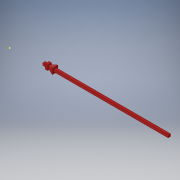
# Autodesk Inventor part: MiddleStick
Saved by Autodesk Inventor 2018.2 (Build 222227000, 227)
## iProperties
Created: 2018-04-10
Part Number: MiddleStick
Material: Generisch
Document SubType Name: Modeling
Designer: Nick Koch
Density: 1 g/cm^3
Appearance: Vorgabe
Author: Nick Koch
Autodesk Inventor part; units mm, degrees
ref_plane "YZ Plane" through (0, 0, 0) normal (1, 0, 0) x (0, 1, 0)
ref_plane "XZ Plane" through (0, 0, 0) normal (0, 1, 0) x (-1, 0, 0)
ref_plane "XY Plane" through (0, 0, 0) normal (0, 0, 1) x (1, 0, 0)
sketch "Skizze4" plane through (0, 0, 0) normal (0, 0, 1) x (1, 0, 0)
  line L0 (0, 0) -> (200, 0)
  line L1 (200, 0) -> (200, 3)
  line L2 (200, 3) -> (0, 3)
  line L3 (0, 3) -> (0, 0)
  dimension "d12" = 200
  dimension "d13" = 3
  constraints: 8 end point, 2 parallel, 1 horizontal, 1 perpendicular
  measures "d12" distance of L2.end L1.end
  measures "d13" distance of L1.end L0.end
extrude "Extrusion4" add sketch "Skizze4" along normal blind 3
sketch "Skizze5" plane through (0, 0, 3) normal (0, 0, 1) x (1, 0, 0)
  line L0 (47, 5) -> (50, 5)
  line L1 (50, 5) -> (50, -2)
  line L2 (50, -2) -> (47, -2)
  line L3 (47, -2) -> (47, 5)
  line L4 (200, 0) -> (200, 3) projected
  line L5 (0, 3) -> (0, 0) projected
  line L6 (200, 3) -> (0, 3) projected
  line L7 (0, 0) -> (200, 0) projected
  dimension "d16" = 150
  dimension "d17" = 47
  dimension "d18" = 2
  dimension "d19" = 2
  constraints: 8 end point, 2 parallel, 1 horizontal, 1 perpendicular
  measures "d16" distance between parallel lines of L4 L1
  measures "d17" distance between parallel lines of L5 L3
  measures "d18" distance between parallel lines of L0 L6
  measures "d19" distance between parallel lines of L7 L2
extrude "Extrusion5" add sketch "Skizze5" along normal blind 2 and the other way blind 5 contours L0 L1 L6 L3 | L6 L1 L7 L3 | L7 L1 L2 L3
sketch "Skizze6" plane through (0, 0, -2) normal (0, 0, -1) x (-1, 0, 0)
  point P0 (0, 0)
sketch "Skizze7" plane through (0, 0, 0) normal (0, 0, -1) x (-1, 0, 0)
  line L0 (-200, 3) -> (-50, 3) projected
  line L1 (-78, 3) -> (-50, 3)
  line L2 (-50, 3) -> (-50, 5)
  line L3 (-50, 5) -> (-78, 5)
  line L4 (-78, 5) -> (-78, 3)
  line L5 (-50, 5) -> (-48, 5)
  line L6 (-48, 5) -> (-48, 33)
  line L7 (-48, 33) -> (-50, 33)
  line L8 (-50, 33) -> (-50, 5)
  line L9 (-50, -2) -> (-50, 5) projected
  arc A0 (-50, 30) -> (-75, 5) centre (-50, 5) ccw
  arc A1 (-50, 27.2) -> (-72.2, 5) centre (-50, 5) ccw
  line L10 (-50, 5) -> (-59.1924, 14.1924)
  line L11 (-50, 5) -> (-37, 5) construction
  circle A2 centre (-59.1924, 14.1924) radius 2.5
  line L12 (-59.1924, 14.1924) -> (-50, 14.1924)
  line L13 (-59.1924, 14.1924) -> (-50, 14.1924)
  line L14 (-50, 14.1924) -> (-50, 13.3924)
  line L15 (-50, 13.3924) -> (-59.1924, 13.3924)
  line L16 (-59.1924, 13.3924) -> (-59.1924, 14.1924)
  line L17 (-50, 14.1924) -> (-59.1924, 14.1924)
  line L18 (-59.1924, 14.1924) -> (-59.1924, 14.9924)
  line L19 (-59.1924, 14.9924) -> (-50, 14.9924)
  line L20 (-50, 14.9924) -> (-50, 14.1924)
  line L21 (-50, 30) -> (-50, 27.2)
  line L22 (-75, 5) -> (-72.2, 5)
  point P0 (0, 0)
  dimension "d24" = 2
  dimension "d25" = 2
  dimension "d26" = 50
  dimension "d27" = 2.8
  dimension "d28" = 13
  dimension "d29" = 135
  dimension "d30" = 5
  dimension "d31" = 0.8
  dimension "d32" = 0.8
  dimension "d33" = 28
  dimension "d34" = 28
  constraints: 42 end point, 8 parallel, 7 perpendicular, 4 point on circle, 4 point on line, 3 centre point, 3 horizontal, 2 coincident, 1 collinear, 1 equal length, 1 vertical
  measures "d24" distance of L2.end L1.end
  measures "d25" distance of L7.end L6.end
  measures "d26" diameter of A0
  measures "d27" radial gap between concentric circles of A0 A1
  measures "d28" distance of L10.start L10.end
  measures "d29" angle of L11 L10
  measures "d30" diameter of A2
  measures "d31" distance of L12.end L14.end
  measures "d32" distance of L12.start L18.end
  measures "d33" distance of L5.end L6.end
  measures "d34" distance of L2.end L3.end
extrude "Extrusion6" add sketch "Skizze7" against normal blind 3 contours L4 L3 L2 L0 | L8 L7 L6 L5 | A0 L8 A1 L3 | L15 A2 L12 L8 | A2 L19 L18 L16 L15 L10 | L10 L15 A2 | L12 A2 L19 L8 | L15 L10 L12 A2 | L15 L16 L10 | A2 L12 L18 L19
sketch "Skizze8" plane through (0, 0, 0) normal (0, 0, -1) x (-1, 0, 0)
  arc A0 (-56.8238, 14.9924) -> (-56.8238, 13.3924) centre (-59.1924, 14.1924) ccw projected
  circle A1 centre (-59.1924, 14.1924) radius 2.5
  line L0 (-56.8238, 13.3924) -> (-50, 13.3924) projected
  line L1 (-56.8238, 13.3924) -> (-50, 13.3924)
  line L2 (-50, 13.3924) -> (-50, 14.9924)
  line L3 (-56.8238, 14.9924) -> (-50, 14.9924) projected
  line L4 (-50, 14.9924) -> (-56.8238, 14.9924)
  point P0 (0, 0)
  constraints: 6 end point, 2 perpendicular, 1 centre point, 1 coincident, 1 collinear
extrude "Extrusion7" cut sketch "Skizze8" against normal blind 0.75 contours L3 L2 L0 A1
sketch "Skizze9" plane through (0, 0, 3) normal (0, 0, 1) x (1, 0, 0)
  arc A0 (56.8238, 13.3924) -> (56.8238, 14.9924) centre (59.1924, 14.1924) ccw projected
  circle A1 centre (59.1924, 14.1924) radius 2.5
  line L0 (50, 14.9924) -> (50, 27.2) projected
  line L1 (56.8238, 14.9924) -> (50, 14.9924)
  line L2 (50, 14.9924) -> (50, 13.3924) projected
  line L3 (50, 14.9924) -> (50, 13.3924)
  line L4 (50, 13.3924) -> (56.8238, 13.3924)
  point P0 (0, 0)
  constraints: 6 end point, 2 perpendicular, 1 coincident, 1 horizontal, 3 other
extrude "Extrusion8" cut sketch "Skizze9" against normal blind 0.75 contours L4 L2 L1 A1
sketch "Skizze10" plane through (0, 0, 0) normal (0, 0, -1) x (-1, 0, 0)
  line L0 (-47, 3) -> (-42, 3)
  line L1 (-47, 3) -> (0, 3) projected
  line L2 (-42, 3) -> (-42, 0)
  line L3 (-47, 3) -> (-47, 0) projected
  line L4 (-42, 0) -> (-47, 0)
  line L5 (-47, 0) -> (-47, 3)
  line L6 (-42, 3) -> (0, 3)
  line L7 (0, 3) -> (0, 0)
  line L8 (0, 0) -> (-42, 0)
  line L9 (-42, 0) -> (-42, 3)
  dimension "d41" = 5
  constraints: 16 end point, 3 equal length, 3 perpendicular, 1 horizontal, 1 point on line
  measures "d41" distance of L0.start L0.end
extrude "Extrusion9" cut sketch "Skizze10" against normal blind 3 contours L1 L7 L8 L2
sketch "Skizze11" plane through (200, 3, 3) normal (0, 1, 0) x (1, 0, 0)
  line L0 (-122, 3) -> (-122, 0) projected
  line L1 (-150, 0) -> (0, 0) projected
  line L2 (0, 0) -> (-122, 0) projected
  line L3 (-122, 0) -> (-117, 0)
  line L4 (-117, 0) -> (-117, 5)
  line L5 (-117, 5) -> (-122, 5)
  line L6 (-122, 5) -> (-122, 0)
  line L7 (-122, 0) -> (-117, 0)
  line L8 (-117, 0) -> (-117, -2)
  line L9 (-117, -2) -> (-122, -2)
  line L10 (-122, -2) -> (-122, 0)
  point P0 (-200, 3)
  dimension "d48" = 5
  dimension "d49" = 5
  dimension "d50" = 2
  constraints: 16 end point, 4 parallel, 2 horizontal, 2 perpendicular, 1 point on line
  measures "d48" distance of L5.end L4.end
  measures "d49" distance of L4.end L3.end
  measures "d50" distance of L7.end L8.end
extrude "Extrusion10" add sketch "Skizze11" along normal blind 2 and the other way blind 5
chamfer "Fase1" distance 5 distance2 2 1 edges at (78, -2, 1.5) measured on face at (78.5, -2, 1.5)
chamfer "Fase2" distance 5 distance2 2 1 edges at (78, 5, -1) measured on face at (78.5, 5, -1)
chamfer "Fase3" distance 5 distance2 2 1 edges at (78, 5, 4) measured on face at (78.5, 5, 4)
chamfer "Fase4" distance 2 distance2 5 1 edges at (78, 1.5, 5) measured on face at (78, 1.5, 4.5)
chamfer "Fase5" distance 5 distance2 2 1 edges at (78, 1.5, -2) measured on face at (78.5, 1.5, -2)
sketch "Skizze13" plane through (0, 0, 0) normal (0, 0, -1) x (-1, 0, 0)
  line L0 (-78, 3) -> (-83, 5) projected
  line L1 (-75, 5) -> (-83, 5) projected
  line L2 (-78, 3) -> (-83, 5)
  line L3 (-83, 5) -> (-78, 5)
  line L4 (-78, 3) -> (-78, 5)
  point P0 (0, 0)
  constraints: 6 end point, 1 perpendicular, 1 point on line
extrude "Extrusion12" cut sketch "Skizze13" against normal blind 5.75
sketch "Skizze14" plane through (48, 5, 0) normal (-1, 0, 0) x (0, 0, 1)
  line L0 (0, 28) -> (3, 28) projected
  line L1 (0, 0) -> (3, 0)
  line L2 (3, 0) -> (3, 28)
  line L3 (3, 28) -> (0, 28)
  line L4 (0, 28) -> (0, 0)
  point P0 (0, -5)
  constraints: 8 end point, 2 parallel, 1 horizontal, 1 perpendicular
extrude "Extrusion13" add sketch "Skizze14" along normal blind 1
offset faces "Größe1" outward -0.2 faces at (52.2746, 14.9924, 1.25)
offset faces "Größe2" outward -0.2 faces at (54.5492, 13.3924, 1.25)
sketch "Skizze16" plane through (0, 0, 0) normal (0, 0, -1) x (-1, 0, 0)
  line L0 (-47, 5) -> (-47, -2) projected
  line L1 (-47, 5) -> (-50, 5) projected
  line L2 (-47, 5) -> (-50, 5)
  line L3 (-78, 5) -> (-75, 5) projected
  line L4 (-50, 5) -> (-78, 5)
  line L5 (-83, 5) -> (-78, 3) projected
  line L6 (-78, 5) -> (-78, 3)
  line L7 (-78, 3) -> (-50, 3)
  line L8 (-50, 0) -> (-50, 5) projected
  line L9 (-47, 33) -> (-47, 5) projected
  line L10 (-47, 5) -> (-47, 33)
  line L11 (-47, 33) -> (-43.9004, 53.8234)
  line L12 (-43.9004, 53.8234) -> (-68.5233, 46.8462)
  line L13 (-68.5233, 46.8462) -> (-80.5, 35.6832)
  line L14 (-80.5, 35.6832) -> (-83, 17.5815)
  line L15 (-78, 5) -> (-78, 3) projected
  line L16 (-83, 17.5815) -> (-78, 5)
  point P0 (0, 0)
  constraints: 20 end point, 3 collinear, 2 perpendicular, 1 point on line
extrude "Extrusion14" cut sketch "Skizze16" against normal blind 10
sketch "Skizze17" plane through (83, -2, 5) normal (1, 0, 0) x (0, 0, -1)
  line L0 (2, 2) -> (0, 0) projected
  line L1 (0, 0) -> (0, 7) projected
  line L2 (0, 0) -> (0, 7)
  line L3 (0, 7) -> (7, 7)
  line L4 (7, 7) -> (7, 0) projected
  line L5 (7, 7) -> (7, 0)
  line L6 (0, 0) -> (7, 0) projected
  line L7 (7, 0) -> (0, 0)
  line L8 (5, 5) -> (2, 5) projected
  line L9 (5, 2) -> (5, 5)
  line L10 (5, 5) -> (2, 5)
  line L11 (2, 5) -> (2, 2)
  line L12 (2, 2) -> (5, 2) projected
  line L13 (2, 2) -> (5, 2)
  constraints: 16 end point, 4 perpendicular, 3 collinear, 1 vertical
extrude "Extrusion15" cut sketch "Skizze17" against normal blind 10
sketch "Skizze18" plane through (50, -2, 5) normal (1, 0, 0) x (0, 0, -1)
  line L0 (0, 7) -> (7, 7) projected
  line L1 (0, 0) -> (0.5, 0)
  line L2 (0.5, 0) -> (0.5, 7)
  line L3 (0.5, 7) -> (0, 7)
  line L4 (0, 7) -> (0, 0)
  line L5 (0, 0) -> (7, 0) projected
  line L6 (7, 0) -> (6.5, 0)
  line L7 (6.5, 0) -> (6.5, 7)
  line L8 (6.5, 7) -> (7, 7)
  line L9 (7, 7) -> (7, 0)
  line L10 (0, 0) -> (7, 0)
  line L11 (7, 0) -> (7, 1)
  line L12 (7, 1) -> (0, 1)
  line L13 (0, 1) -> (0, 0)
  line L14 (7, 7) -> (7, 0) projected
  line L15 (0, 7) -> (7, 7)
  line L16 (7, 7) -> (7, 6)
  line L17 (7, 6) -> (0, 6)
  line L18 (0, 6) -> (0, 7)
  point P0 (5, 2)
  dimension "d83" = 0.5
  dimension "d84" = 0.5
  dimension "d85" = 7
  dimension "d86" = 1
  dimension "d87" = 1
  constraints: 32 end point, 8 parallel, 4 horizontal, 4 perpendicular, 3 point on line
  measures "d83" distance of L3.end L2.end
  measures "d84" distance of L7.end L8.end
  measures "d85" distance of L12.end L11.end
  measures "d86" distance of L11.end L10.end
  measures "d87" distance of L15.end L16.end
extrude "Extrusion16" cut sketch "Skizze18" against normal blind 10 contours L0 L2 L17 L4 | L0 L7 L17 L2 | L17 L2 L12 L4 | L0 L9 L17 L7 | L12 L2 L1 L4 | L17 L9 L12 L7 | L12 L7 L5 L2 | L12 L9 L5 L7
move faces "Verschieben1" translate (-1, 0, 0) faces at (47, 1, 4)
move faces "Verschieben2" translate (-1, 0, 0) faces at (50, 1, 4)
sketch "Skizze19" plane through (49, 0, 0) normal (0, -1, 0) x (1, 0, 0)
  line L0 (0, -1.5) -> (7, -1.5)
  line L1 (7, -1.5) -> (7, 4.5)
  line L2 (7, 4.5) -> (0, 4.5)
  line L3 (0, 4.5) -> (0, -1.5)
  point P0 (-49, 0)
  dimension "d96" = 7
  constraints: 8 end point, 2 parallel, 1 horizontal, 1 perpendicular
  measures "d96" distance of L2.end L1.end
extrude "Extrusion17" add sketch "Skizze19" along normal blind 2
sketch "Skizze20" plane through (46, -1, 4.5) normal (0, 0, 1) x (1, 0, 0)
  line L0 (10, 1) -> (10, -1) projected
  line L1 (10, -1) -> (3, 1)
  line L2 (10, 1) -> (3, 1) projected
  line L3 (3, 1) -> (10, 1)
  line L4 (10, 1) -> (10, -1)
  line L5 (3, 1) -> (3, 4) projected
  line L6 (10, -1) -> (3, -1) projected
  line L7 (3, 1) -> (3, -1)
  line L8 (3, -1) -> (10, -1)
  line L9 (10, -1) -> (3, 1)
  point P0 (-46, 1)
  constraints: 12 end point, 2 perpendicular, 1 collinear, 1 vertical
extrude "Extrusion18" cut sketch "Skizze20" against normal blind 9.25 contours L6 L7 L1
sketch "Skizze21" plane through (0, 0, 3) normal (0, 0, 1) x (1, 0, 0)
  line L0 (49, 4) -> (56, 4)
  line L1 (56, 4) -> (56, -4.0594)
  line L2 (56, -4.0594) -> (49, -4.0594)
  line L3 (49, -4.0594) -> (49, 4)
  point P0 (0, 0)
  dimension "d101" = 7
  constraints: 8 end point, 2 parallel, 1 horizontal, 1 perpendicular
  measures "d101" distance of L1.end L2.end
extrude "Extrusion19" add sketch "Skizze21" along normal blind 2
sketch "Skizze22" plane through (49, -4.0594, 3) normal (0, -1, 0) x (1, 0, 0)
  line L0 (0, 2) -> (7, 2) projected
  line L1 (0, 0) -> (0, 2) projected
  line L2 (7, 2) -> (0, 0)
  line L3 (0, 0) -> (0, 2)
  line L4 (0, 1.5) -> (-3, 1.5) projected
  line L5 (0, 2) -> (7, 2)
  point P0 (-49, -3)
  constraints: 6 end point, 2 perpendicular
extrude "Extrusion20" cut sketch "Skizze22" against normal blind 14.75
sketch "Skizze23" plane through (0, 0, 3) normal (0, 0, -1) x (-1, 0, 0)
  line L0 (-49, 0) -> (-49, -1) projected
  line L1 (-56, -2) -> (-49, 0) projected
  line L2 (-49, 0) -> (-56, -2)
  line L3 (-56, -4.0594) -> (-49, -4.0594) projected
  line L4 (-56, -2) -> (-56, -4.0594)
  line L5 (-56, -4.0594) -> (-49, -4.0594)
  line L6 (-49, -4.0594) -> (-49, 0)
  point P0 (0, 0)
  constraints: 8 end point, 2 collinear, 2 perpendicular
extrude "Extrusion21" cut sketch "Skizze23" against normal blind 13.75
sketch "Skizze24" plane through (49, 3, 0) normal (0, 1, 0) x (1, 0, 0)
  line L0 (0, 4.1822) -> (7, 4.1822)
  line L1 (7, 4.1822) -> (7, -9.8185)
  line L2 (7, -9.8185) -> (0, -9.8185)
  line L3 (0, -9.8185) -> (0, 4.1822)
  point P0 (-49, 0)
  dimension "d108" = 7
  constraints: 8 end point, 2 parallel, 1 horizontal, 1 perpendicular
  measures "d108" distance of L1.end L2.end
extrude "Extrusion22" add sketch "Skizze24" along normal blind 2
sketch "Skizze25" plane through (49, 3, 9.8185) normal (0, 0, 1) x (1, 0, 0)
  line L0 (0, 0) -> (7, 2)
  line L1 (7, 0) -> (7, 2) projected
  line L2 (7, 2) -> (7, 0)
  line L3 (7, 0) -> (0, 0)
  line L4 (0, 0) -> (0, 2) projected
  line L5 (7, 2) -> (0, 2)
  line L6 (0, 2) -> (0, 0)
  line L7 (0, 0) -> (7, 2)
  point P0 (-49, -3)
  constraints: 12 end point, 2 perpendicular, 1 collinear, 1 horizontal
extrude "Extrusion23" cut sketch "Skizze25" against normal blind 50.25 contours L4 L5 L0
sketch "Skizze26" plane through (0, 0, 0) normal (0, 0, -1) x (-1, 0, 0)
  line L0 (-49, -1) -> (-56, -1)
  line L1 (-56, -1) -> (-56, 5.8181)
  line L2 (-56, 5.8181) -> (-49, 5.8181)
  line L3 (-49, 5.8181) -> (-49, -1)
  point P0 (0, 0)
  dimension "d113" = 7
  constraints: 8 end point, 2 parallel, 1 horizontal, 1 perpendicular
  measures "d113" distance of L1.end L2.end
extrude "Extrusion24" add sketch "Skizze26" along normal blind 2
sketch "Skizze27" plane through (56, 5, -2) normal (-0.2747211, 0.9615239, 0) x (0.9615239, 0.2747211, 0)
  line L0 (-7.2801, 0) -> (0, 0) projected
  line L1 (-7.2801, 2.1822) -> (0, 2.1822) projected
  line L2 (0, 0) -> (0, 2.1822)
  line L3 (0, 2.1822) -> (-7.2801, 2.1822)
  line L4 (-7.2801, 0) -> (-6.5059, 0) projected
  line L5 (-7.2801, 2.1822) -> (-7.2801, 0)
  line L6 (0, 0) -> (0, 2.1822) projected
  line L7 (-7.2801, 0) -> (0, 0)
  point P0 (-55.2189, -2)
  constraints: 8 end point, 2 perpendicular, 1 collinear, 1 vertical
extrude "Extrusion25" cut sketch "Skizze27" against normal blind 7
sketch "Skizze28" plane through (49, 5.8181, 0) normal (0, 1, 0) x (1, 0, 0)
  line L0 (0, 0) -> (0, 2) projected
  line L1 (7, 2) -> (0, 0)
  line L2 (0, 0) -> (0, 2)
  line L3 (0, 0) -> (3.5, 0) projected
  line L4 (0, 2) -> (7, 2)
  point P0 (-49, 0)
  constraints: 6 end point, 2 perpendicular
extrude "Extrusion26" cut sketch "Skizze28" against normal blind 16.5
sketch "Skizze29" plane through (0, 0, 0) normal (0, 0, 1) x (1, 0, 0)
  line L0 (56, 5) -> (49, 3) projected
  line L1 (56, 5) -> (49, 3)
  line L2 (56, 5.8181) -> (49, 5.8181) projected
  line L3 (49, 3) -> (49, 5.8181)
  line L4 (49, 5.8181) -> (56, 5.8181)
  line L5 (56, 5.8181) -> (56, 5)
  point P0 (0, 0)
  constraints: 8 end point, 2 perpendicular, 1 collinear
extrude "Extrusion27" cut sketch "Skizze29" against normal blind 19.75
sketch "Skizze30" plane through (49, 3, 0) normal (0, -1, 0) x (1, 0, 0)
  line L0 (0, 3) -> (0, 0) projected
  line L1 (7, 5) -> (0, 3) projected
  line L2 (0, 3) -> (7, 5)
  line L3 (7, 5) -> (7, 9.8185) projected
  line L4 (7, 5) -> (7, 9.8185)
  line L5 (0, 9.8185) -> (0, 4.5) projected
  line L6 (7, 9.8185) -> (0, 9.8185)
  line L7 (0, 9.8185) -> (0, 3)
  point P0 (-49, 0)
  constraints: 8 end point, 3 collinear, 1 perpendicular
extrude "Extrusion28" cut sketch "Skizze30" against normal blind 12.5
move faces "Verschieben3" translate (0, -1, 0) faces at (55.4167, -1, -1.6667)
sketch "Skizze31" plane through (54.25, -2, -1.5) normal (0, 0, 1) x (1, 0, 0)
  line L0 (0, 0.5) -> (0, 0) projected
  line L1 (0, 0.5) -> (0, 0)
  line L2 (1.75, 0) -> (0, 0.5) projected
  line L3 (0, 0) -> (1.75, 0)
  line L4 (1.75, 0) -> (0, 0.5)
  point P0 (-54.25, 2)
  constraints: 6 end point, 2 collinear, 1 perpendicular
extrude "Extrusion29" cut sketch "Skizze31" against normal blind 3
sketch "Skizze32" plane through (0, 0, 0) normal (0, 0, 1) x (1, 0, 0)
  line L0 (49, 0) -> (52.5, -1) projected
  line L1 (49, -1) -> (49, 0) projected
  line L2 (49, 0) -> (49, -1)
  line L3 (49, -1) -> (52.5, -1)
  line L4 (52.5, -1) -> (49, 0)
  point P0 (0, 0)
  constraints: 6 end point, 1 collinear, 1 perpendicular
extrude "Extrusion30" cut sketch "Skizze32" against normal blind 1
